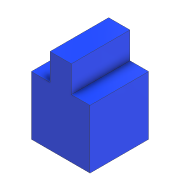
# Autodesk Inventor part: Agarose-block
Saved by Autodesk Inventor 2021 (Build 250183000, 183)
## iProperties
Created: 2023-03-07
Part Number: Agarose-block
Material: Generic
Document SubType Name: Modeling
Designer: nvladi
Density: 1 g/cm^3
Appearance: Default
Author: nvladi
Autodesk Inventor part; units mm, degrees
ref_plane "YZ Plane" through (0, 0, 0) normal (1, 0, 0) x (0, 1, 0)
ref_plane "XZ Plane" through (0, 0, 0) normal (0, 1, 0) x (-1, 0, 0)
ref_plane "XY Plane" through (0, 0, 0) normal (0, 0, 1) x (1, 0, 0)
sketch "Sketch1" plane through (0, 0, 0) normal (0, 0, 1) x (1, 0, 0)
  line L0 (2.75, -2.75) -> (-2.75, -2.75)
  line L1 (-2.75, -2.75) -> (-2.75, 2.75)
  line L2 (-2.75, 2.75) -> (2.75, 2.75)
  line L3 (2.75, 2.75) -> (2.75, -2.75)
  line L4 (2.75, -2.75) -> (-2.75, 2.75) construction
  line L5 (-2.75, -2.75) -> (2.75, 2.75) construction
  line L6 (1, 0.25) -> (1, 5.25)
  line L7 (1, 5.25) -> (-1, 5.25)
  line L8 (-1, 5.25) -> (-1, 0.25)
  line L9 (-1, 0.25) -> (1, 0.25)
  line L10 (1, 0.25) -> (-1, 5.25) construction
  line L11 (1, 5.25) -> (-1, 0.25) construction
  point P0 (0, 0)
  point P1 (0, 2.75)
  point P2 (-1, 2.75)
  point P3 (1, 2.75)
  dimension "d0" = 5.5
  dimension "d1" = 5.5
  dimension "d2" = 2
  dimension "d3" = 5
  constraints: 24 end point, 5 midpoint, 4 parallel, 2 perpendicular, 1 horizontal, 1 vertical
  measures "d0" distance of L1.end L2.end
  measures "d1" distance of L0.end L1.end
  measures "d2" distance of L7.end L6.end
  measures "d3" distance between parallel lines of L9 L7
extrude "Extrusion1" add sketch "Sketch1" along normal blind 5.5
body "Solid1"
